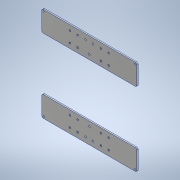
# Autodesk Inventor part: BedCarriageA
Saved by Autodesk Inventor 2020.2 (Build 242310000, 310)
## iProperties
Created: 2017-10-23
Part Number: BedCarriageA
Material: Aluminium 6061
Document SubType Name: Modeling
Designer: Haras
Density: 2.7 g/cm^3
Appearance: Aluminium — płaski
Author: Haras
Autodesk Inventor part; units mm, degrees
ref_plane "YZ Plane" through (0, 0, 0) normal (1, 0, 0) x (0, 1, 0)
ref_plane "XZ Plane" through (0, 0, 0) normal (0, 1, 0) x (-1, 0, 0)
ref_plane "XY Plane" through (0, 0, 0) normal (0, 0, 1) x (1, 0, 0)
sketch "Szkic1" plane through (0, 0, 0) normal (0, 1, 0) x (-1, 0, 0)
  line L0 (110, 109.5) -> (-110, 109.5)
  line L1 (-110, 109.5) -> (-110, 61.5)
  line L2 (110, 61.5) -> (110, 109.5)
  line L3 (-110, -61.5) -> (-110, -109.5)
  line L4 (-110, -109.5) -> (110, -109.5)
  line L5 (110, -109.5) -> (110, -61.5)
  line L6 (110, 0) -> (-110, 0) construction
  line L7 (0, 61) -> (0, -61) construction
  line L8 (15, 61.5) -> (15, -61.5)
  line L9 (-15, 61.5) -> (-15, -61.5)
  line L10 (-110, 61.5) -> (-15, 61.5)
  line L11 (15, 61.5) -> (110, 61.5)
  line L12 (110, -61.5) -> (15, -61.5)
  line L13 (-15, -61.5) -> (-110, -61.5)
  point P0 (0, 0)
  point P1 (110, -85.5)
  point P2 (-110, -85.5)
  dimension "d0" = 48
  dimension "d2" = 220
  dimension "d3" = 30
  dimension "d4" = 123
  constraints: 28 end point, 7 perpendicular, 6 parallel, 4 horizontal, 4 midpoint, 3 collinear, 2 point on line, 2 vertical alignment, 3 other
  measures "d0" distance of L2.start L0.start
  measures "d2" distance of L3.end L4.end
  measures "d3" distance between parallel lines of L9 L8
  measures "d4" distance between parallel lines of L12 L11
extrude "Wyciągnięcie proste1" add sketch "Szkic1" along normal blind 3
sketch "Szkic2" plane through (0, 3, 0) normal (0, 1, 0) x (1, 0, 0)
  line L0 (-110, -109.5) -> (110, -109.5) projected
  line L1 (0, -109.5) -> (0, 109.5) construction
  line L2 (110, 109.5) -> (-110, 109.5) projected
  line L3 (-15, 61.5) -> (-15, -61.5) projected
  line L4 (-15, 0) -> (15, 0) construction
  line L5 (15, -61.5) -> (15, 61.5) projected
  line L6 (-110, -61.5) -> (-110, -109.5) projected
  line L7 (110, -109.5) -> (110, -61.5) projected
  line L8 (-15, -61.5) -> (-110, -61.5) projected
  point P0 (0, 0)
  point P1 (-45, -72.5)
  point P2 (-45, -97.5)
  point P3 (-27, -97.5)
  point P4 (-27, -72.5)
  point P5 (-45, 72.5)
  point P6 (-45, 97.5)
  point P7 (-27, 97.5)
  point P8 (-27, 72.5)
  point P9 (45, -72.5)
  point P10 (45, -97.5)
  point P11 (27, -97.5)
  point P12 (27, -72.5)
  point P13 (45, 72.5)
  point P14 (27, 72.5)
  point P15 (27, 97.5)
  point P16 (45, 97.5)
  dimension "d8" = 25
  dimension "d9" = 18
  dimension "d10" = 12
  dimension "d19" = 11
  constraints: 12 symmetric about line, 4 end point, 4 midpoint, 2 horizontal alignment, 2 vertical alignment
  measures "d8" distance of point (-45, -97.5) point (-45, -72.5)
  measures "d9" distance of point (-27, -72.5) point (-45, -72.5)
  measures "d10" distance from line of L3 point (-27, -72.5)
  measures "d19" distance from line of L8 point (-45, -72.5)
hole "Otwór1" at (-45, 3, 72.5) at (-45, 3, 97.5) at (-27, 3, 97.5) at (-27, 3, 72.5) at (-45, 3, -72.5) at (-27, 3, -72.5) at (-27, 3, -97.5) at (-45, 3, -97.5) at (45, 3, 97.5) at (45, 3, 72.5) at (27, 3, 72.5) at (27, 3, 97.5) at (45, 3, -72.5) at (45, 3, -97.5) at (27, 3, -97.5) at (27, 3, -72.5) direction (0, -1, 0) diameter 4 end through all
fillet "Zaokrąglenie1" radius 3 12 edges at (-110, 1.5, 109.5) (-110, 1.5, 61.5) (-110, 1.5, -61.5) (-110, 1.5, -109.5) (110, 1.5, 109.5) (110, 1.5, 61.5) (110, 1.5, -109.5) (110, 1.5, -61.5) (15, 1.5, -61.5) (15, 1.5, 61.5) (-15, 1.5, 61.5) (-15, 1.5, -61.5)
sketch "Szkic3" plane through (0, 0, 0) normal (0, -1, 0) x (1, 0, 0)
  arc A0 (-107, 109.5) -> (-110, 106.5) centre (-107, 106.5) ccw projected
  arc A1 (-110, -106.5) -> (-107, -109.5) centre (-107, -106.5) ccw projected
  arc A2 (107, -109.5) -> (110, -106.5) centre (107, -106.5) ccw projected
  arc A3 (110, 106.5) -> (107, 109.5) centre (107, 106.5) ccw projected
  line L0 (-107, 109.5) -> (107, 109.5) projected
  line L1 (110, 106.5) -> (110, 64.5) projected
  line L2 (107, -109.5) -> (-107, -109.5) projected
  line L3 (-110, -106.5) -> (-110, -64.5) projected
  point P0 (0, 0)
  point P1 (-105, -104.5)
  point P2 (-105, 104.5)
  point P3 (105, 104.5)
  point P4 (105, -104.5)
  dimension "d29" = 5
  dimension "d30" = 5
  dimension "d31" = 5
  dimension "d32" = 5
  constraints: 2 horizontal alignment, 2 vertical alignment
  measures "d29" distance from line of L0 point (105, 104.5)
  measures "d30" distance from line of L1 point (105, 104.5)
  measures "d31" distance from line of L2 point (-105, -104.5)
  measures "d32" distance from line of L3 point (-105, -104.5)
hole "Otwór3" at (-105, 0, -104.5) at (-105, 0, 104.5) at (105, 0, 104.5) at (105, 0, -104.5) direction (0, 1, 0) diameter 3 end through all
sketch "Szkic4" plane through (0, 0, 0) normal (0, -1, 0) x (1, 0, 0)
  line L0 (15, 58.5) -> (15, -58.5) projected
  line L1 (15, 0) -> (-15, 0) construction
  line L2 (-15, -58.5) -> (-15, 58.5) projected
  line L3 (-107, 109.5) -> (107, 109.5) projected
  line L4 (0, 109.5) -> (0, -109.5) construction
  line L5 (107, -109.5) -> (-107, -109.5) projected
  point P0 (0, 0)
  point P1 (9, 5.5)
  point P2 (9, -5.5)
  point P3 (-9, -5.5)
  point P4 (-9, 5.5)
  dimension "d40" = 11
  dimension "d41" = 18
  constraints: 4 end point, 4 midpoint, 2 horizontal alignment, 2 symmetric about line, 2 vertical alignment
  measures "d40" distance of point (9, -5.5) point (9, 5.5)
  measures "d41" distance of point (-9, -5.5) point (9, -5.5)
hole "Otwór4" at (9, 0, 5.5) at (9, 0, -5.5) at (-9, 0, -5.5) at (-9, 0, 5.5) direction (0, 1, 0) diameter 4 end through all
thread "Gwint1" size "M4x0.7" class "6H" standard "ANSI Metric M Profile" full length
thread "Gwint2" size "M4x0.7" class "6H" standard "ANSI Metric M Profile" full length
thread "Gwint3" size "M4x0.7" class "6H" standard "ANSI Metric M Profile" full length
thread "Gwint4" size "M4x0.7" class "6H" standard "ANSI Metric M Profile" full length
thread "Gwint5" size "M4x0.7" class "6H" standard "ANSI Metric M Profile" full length
thread "Gwint6" size "M4x0.7" class "6H" standard "ANSI Metric M Profile" full length
thread "Gwint7" size "M4x0.7" class "6H" standard "ANSI Metric M Profile" full length
thread "Gwint8" size "M4x0.7" class "6H" standard "ANSI Metric M Profile" full length
thread "Gwint9" size "M4x0.7" class "6H" standard "ANSI Metric M Profile" full length
thread "Gwint10" size "M4x0.7" class "6H" standard "ANSI Metric M Profile" full length
thread "Gwint11" size "M4x0.7" class "6H" standard "ANSI Metric M Profile" full length
thread "Gwint12" size "M4x0.7" class "6H" standard "ANSI Metric M Profile" full length
thread "Gwint13" size "M4x0.7" class "6H" standard "ANSI Metric M Profile" full length
thread "Gwint14" size "M4x0.7" class "6H" standard "ANSI Metric M Profile" full length
thread "Gwint15" size "M4x0.7" class "6H" standard "ANSI Metric M Profile" full length
thread "Gwint16" size "M4x0.7" class "6H" standard "ANSI Metric M Profile" full length
thread "Gwint17" size "M4x0.7" class "6H" standard "ANSI Metric M Profile" full length
thread "Gwint18" size "M4x0.7" class "6H" standard "ANSI Metric M Profile" full length
thread "Gwint19" size "M4x0.7" class "6H" standard "ANSI Metric M Profile" full length
thread "Gwint20" size "M4x0.7" class "6H" standard "ANSI Metric M Profile" full length
thread "Gwint21" size "M3x0.5" class "6H" standard "ANSI Metric M Profile" full length
thread "Gwint22" size "M3x0.5" class "6H" standard "ANSI Metric M Profile" full length
thread "Gwint23" size "M3x0.5" class "6H" standard "ANSI Metric M Profile" full length
thread "Gwint24" size "M3x0.5" class "6H" standard "ANSI Metric M Profile" full length
sketch "Sketch5" plane through (0, 0, 0) normal (0, -1, 0) x (1, 0, 0)
  line L0 (-18, 61.5) -> (-107, 61.5) projected
  arc A0 (15, -58.5) -> (18, -61.5) centre (18, -58.5) ccw projected
  line L1 (-18, 61.5) -> (18, 61.5)
  line L2 (18, 61.5) -> (18, -61.5)
  line L3 (18, -61.5) -> (-18, -61.5)
  line L4 (-18, -61.5) -> (-18, 61.5)
  point P0 (0, 0)
  constraints: 8 end point, 2 parallel, 1 horizontal, 1 perpendicular
extrude "Extrusion2" cut sketch "Sketch5" against normal blind 10
sketch "Sketch6" plane through (0, 0, 0) normal (0, -1, 0) x (1, 0, 0)
  circle A0 centre (-8.5, 97.5) radius 2
  circle A1 centre (8.5, 97.5) radius 2
  circle A2 centre (0, 72.5) radius 2
  circle A3 centre (0, -72.5) radius 2
  circle A4 centre (8.5, -97.5) radius 2
  circle A5 centre (-8.5, -97.5) radius 2
  circle A6 centre (45, 72.5) radius 2 projected
  circle A7 centre (27, -72.5) radius 2 projected
  point P0 (0, 0)
  dimension "d99" = 17
  dimension "d100" = 4
  dimension "d101" = 8.5
  dimension "d102" = 25
  dimension "d103" = 25
  constraints: 6 centre point, 5 equal radius, 4 horizontal alignment, 3 vertical alignment
  measures "d99" distance of A1.centre A0.centre
  measures "d100" diameter of A1
  measures "d101" horizontal distance of A1.centre point (0, 0)
  measures "d102" vertical distance of A2.centre A1.centre
  measures "d103" vertical distance of A3.centre A4.centre
extrude "Extrusion3" cut sketch "Sketch6" against normal blind 10 contours A0 | A1 | A2 | A3 | A4 | A5
sketch "Sketch7" plane through (0, 0, 0) normal (0, -1, 0) x (1, 0, 0)
  circle A0 centre (105, 104.5) radius 1.5 projected
  circle A1 centre (105, -104.5) radius 1.5 projected
  circle A2 centre (-105, -104.5) radius 1.5 projected
  circle A3 centre (-105, 104.5) radius 1.5 projected
  point P0 (0, 0)
extrude "Extrusion4" add sketch "Sketch7" against normal up to surface (3 mm away)
sketch "Sketch8" plane through (0, 0, 0) normal (0, -1, 0) x (1, 0, 0)
  circle A0 centre (106, -105.5) radius 1.5
  circle A1 centre (106, 105.5) radius 1.5
  circle A2 centre (-106, -105.5) radius 1.5
  circle A3 centre (-106, 105.5) radius 1.5
  line L0 (107, -109.5) -> (-107, -109.5) projected
  line L1 (110, -64.5) -> (110, -106.5) projected
  line L2 (-107, 109.5) -> (107, 109.5) projected
  line L3 (110, 106.5) -> (110, 64.5) projected
  line L4 (-110, -106.5) -> (-110, -64.5) projected
  point P0 (0, 0)
  dimension "d108" = 3
  dimension "d109" = 4
  dimension "d110" = 4
  dimension "d111" = 4
  dimension "d112" = 4
  dimension "d113" = 4
  constraints: 4 centre point, 3 equal radius, 2 horizontal alignment, 1 vertical alignment
  measures "d108" diameter of A0
  measures "d109" distance from line of L0 A0.centre
  measures "d110" distance from line of L1 A0.centre
  measures "d111" distance from line of L2 A1.centre
  measures "d112" distance from line of L3 A1.centre
  measures "d113" distance from line of L4 A2.centre
extrude "Extrusion5" cut sketch "Sketch8" against normal blind 10
